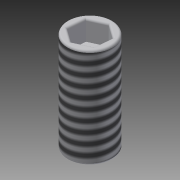
# Autodesk Inventor part: 4_40_hex_cap_screw
Saved by Autodesk Inventor 2014 (Build 180170000, 170)
## iProperties
Created: 2014-03-24
Part Number: 4_40_hex_cap_screw
Material: Generic
Document SubType Name: Modeling
Designer: stephenholtz
Density: 1 g/cm^3
Appearance: Default
Mass: 0.036343 g
Surface Area: 0.764466 cm^2
Volume: 0.036343 cm^3
Author: stephenholtz
Autodesk Inventor part; units mm, degrees
ref_plane "YZ Plane" through (0, 0, 0) normal (1, 0, 0) x (0, 1, 0)
ref_plane "XZ Plane" through (0, 0, 0) normal (0, 1, 0) x (-1, 0, 0)
ref_plane "XY Plane" through (0, 0, 0) normal (0, 0, 1) x (1, 0, 0)
sketch "Sketch4" plane through (0, 0, 0) normal (0, 1, 0) x (-1, 0, 0)
  circle A0 centre (0, 0) radius 1.4224
  dimension "d14" = 2.8448
  constraints: 1 centre point, 1 coincident
  measures "d14" diameter of A0
extrude "Extrusion4" add sketch "Sketch4" along normal blind 6.35
thread "Thread2" size "4-40 UNC" class "2A" standard "ANSI Unified Screw Threads" full length
fillet "Fillet1" radius 0.127 1 edges at (1.4224, 0, 0)
sketch "Sketch5" plane through (0, 6.35, 0) normal (0, 1, 0) x (1, 0, 0)
  line L0 (-0.8884, 0.635) -> (0.1057, 1.0869)
  line L1 (0.1057, 1.0869) -> (0.9941, 0.4519)
  line L2 (0.9941, 0.4519) -> (0.8884, -0.635)
  line L3 (0.8884, -0.635) -> (-0.1057, -1.0869)
  line L4 (-0.1057, -1.0869) -> (-0.9941, -0.4519)
  line L5 (-0.9941, -0.4519) -> (-0.8884, 0.635)
  point P0 (0, 0)
  point P1 (0, 0)
  dimension "d20" = 1.27
  constraints: 12 end point, 1 coincident, 13 other
  measures "d20" vertical distance of L0.start L2.end
extrude "Extrusion5" cut sketch "Sketch5" against normal blind 1.27
fillet "Fillet2" radius 0.127 1 edges at (1.4224, 6.35, 0)
fillet "Fillet3" radius 0.127 6 edges at (0.5499, 6.35, -0.7694) (0.9412, 6.35, 0.0916) (0.3913, 6.35, 0.8609) (-0.5499, 6.35, 0.7694) (-0.9412, 6.35, -0.0916) (-0.3913, 6.35, -0.8609)
body "Solid2"
